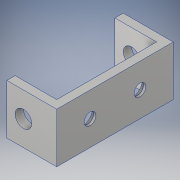
# Autodesk Inventor part: CAR_045_NewCarouselTensioner1.75UChannel
Saved by Autodesk Inventor 2018 (Build 220112000, 112)
## iProperties
Created: 2020-02-15
Part Number: CAR_045_NewCarouselTensioner1.75UChannel
Material: Aluminum 6061
Document SubType Name: Modeling
Designer: user
Mass: 27.6532 g
Surface Area: 74.1934 cm^2
Volume: 10.2419 cm^3
Density: 2.7 g/cm^3
Appearance: Aluminum - Flat
Author: user
Autodesk Inventor part; units mm, degrees
ref_plane "YZ Plane" through (0, 0, 0) normal (1, 0, 0) x (0, 1, 0)
ref_plane "XZ Plane" through (0, 0, 0) normal (0, 1, 0) x (-1, 0, 0)
ref_plane "XY Plane" through (0, 0, 0) normal (0, 0, 1) x (1, 0, 0)
sketch "Sketch1" plane through (0, 0, 0) normal (0, 1, 0) x (-1, 0, 0)
  line L0 (0, 0) -> (19.05, 0)
  line L1 (19.05, 0) -> (19.05, -3.175)
  line L2 (19.05, -3.175) -> (0, -3.175)
  line L3 (0, -3.175) -> (0, 0)
  line L4 (0, 0) -> (3.175, 0)
  line L5 (3.175, 0) -> (3.175, -44.45)
  line L6 (3.175, -44.45) -> (0, -44.45)
  line L7 (0, -44.45) -> (0, 0)
  line L8 (0, -44.45) -> (19.05, -44.45)
  line L9 (19.05, -44.45) -> (19.05, -41.275)
  line L10 (19.05, -41.275) -> (0, -41.275)
  line L11 (0, -41.275) -> (0, -44.45)
  dimension "d0" = 19.05
  dimension "d1" = 3.175
  dimension "d2" = 3.175
  dimension "d3" = 44.45
  dimension "d4" = 19.05
  dimension "d5" = 3.175
  constraints: 24 end point, 6 parallel, 3 horizontal, 3 perpendicular
  measures "d0" distance of L1.end L2.end
  measures "d1" distance of L0.end L1.end
  measures "d2" distance of L5.end L6.end
  measures "d3" distance of L4.end L5.end
  measures "d4" distance of L10.end L9.end
  measures "d5" distance of L9.end L8.end
extrude "Extrusion1" add sketch "Sketch1" along normal blind 19.05
sketch "Sketch2" plane through (-19.05, 0, 0) normal (0, 0, 1) x (1, 0, 0)
  line L0 (0, 0) -> (0, 19.05) projected
  line L1 (0, 0) -> (19.05, 0) projected
  line L2 (19.05, 0) -> (19.05, 19.05) projected
  point P0 (6.35, 9.525)
  dimension "d9" = 19.05
  dimension "d10" = 9.525
  dimension "d18" = 12.7
  measures "d9" distance of L0.start L0.end
  measures "d10" distance from line of L1 point (6.35, 9.525)
  measures "d18" distance from line of point (6.35, 9.525) L2
hole "Hole1" at (-12.7, 9.525, 0) direction (0, 0, -1) diameter 6.35 end through all
sketch "Sketch3" plane through (-3.175, 0, -41.275) normal (-1, 0, 0) x (0, 0, 1)
  line L0 (0, 19.05) -> (38.1, 19.05) projected
  line L1 (0, 0) -> (38.1, 0) projected
  line L2 (38.1, 0) -> (38.1, 19.05) projected
  line L3 (0, 0) -> (0, 19.05) projected
  point P0 (41.275, 0)
  point P1 (9.525, 9.525)
  point P2 (28.575, 9.525)
  dimension "d19" = 9.525
  dimension "d20" = 19.05
  dimension "d21" = 9.525
  dimension "d22" = 9.525
  dimension "d23" = 9.525
  measures "d19" distance from line of L0 point (9.525, 9.525)
  measures "d20" distance between parallel lines of L0 L1
  measures "d21" distance from line of L0 point (28.575, 9.525)
  measures "d22" distance from line of L2 point (28.575, 9.525)
  measures "d23" distance from line of L3 point (9.525, 9.525)
hole "Hole2" at (-3.175, 9.525, -31.75) at (-3.175, 9.525, -12.7) direction (1, 0, 0) diameter 4.4958 end through all countersink diameter 8.4328 countersink angle 82 clearance for "Flat Head Machine Screw (82)" size "#8" standard "Ansi Unified Screw Threads"
equation "\"d4\" = d0"
equation "\"d10\" = 0.5 * d9"
equation "\"d19\" = 0.5 * d20"
equation "\"d21\" = d19"
body "Solid1"
